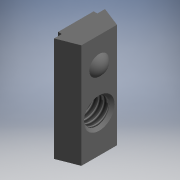
# Autodesk Inventor part: HNTP5-5_app
Saved by Autodesk Inventor 2017.3 (Build 213256000, 256)
## iProperties
Part Number: HNTP5-5_app
Material: Generic
Catalog Web Link: www.cadenas.de
Description: HNTP, HNTPV, HNTPZ, SHNTP_app-Post-Assembly Fitting Spring Nuts For Aluminum Frames
Vendor: MISUMI
Document SubType Name: Modeling
Designer: partserver
Manufacturer: MISUMI
Mass: 0.392555 g
Surface Area: 4.47403 cm^2
Volume: 0.392555 cm^3
Density: 1 g/cm^3
Appearance: PSOLRGB-128-128-128
Category: PARTsolutions
Company: MISUMI
Title: HNTP5-5
Author: Cadenas PARTsolutions
Comments: Post-Assembly Fitting Spring Nuts For Aluminum Frames
PSOL_IDENT_0: {$CADENAS_DATA\23d-libs\misumi\metric\38_al_extrusions_blackets\nuts\shntp.prj},188 {VTYP=3D},{NB=HN
PSOL_IDENT_1: TP5-5_app},{LINA=HNTP5-5},{NN=HNTP, HNTPV, HNTPZ, SHNTP_app},{DATE=28.07.2021 09:30:14},{GEOMDATE=07
PSOL_IDENT_2: .03.2017 06:48:08},{VERSION=},{LINEID=10},{WBVAR=MATB,M},{WBNUMERIC=M}  {NB=HNTP5-5_app},{LINA=HNTP5
PSOL_IDENT_3: -5},{KT=DUMMY},{PN=HNTP5-5},{MATB=HNTP},{MATBALL=304 Stainless Steel},{MATS=SWP-A},{ST=Trivalent Chr
PSOL_IDENT_4: omate},{NO=5},{M=5},{MALG=3,4,5},{AFS=HFS5},{A=5.8},{B=8.3},{E=3.2},{T=3.8},{L=17},{L1=6.0},{TT=6.8}
PSOL_IDENT_5: ,{L11=4}
NB: HNTP5-5_app
NN: HNTP, HNTPV, HNTPZ, SHNTP_app
NT: Post-Assembly Fitting Spring Nuts For Aluminum Frames
NBSYN: $PN._app
LINA: HNTP5-5
CATALOG: Misumi
PN: HNTP5-5
MATB: 1010 Carbon Steel Equivalent
MATBALL: 304 Stainless Steel
MATS: SWP-A
ST: Trivalent Chromate Plating
NO: 5
M: 5
A: 5.8
B: 8.3
E: 3.2
T: 3.8
L: 17
L1: 6
TT: 6.8
SUPPLIER: MISUMI
ARTICLENO: HNTP5-5_app
BOMINFO: HNTP5-5
CREATOR: CADENAS GmbH
Autodesk Inventor part; units mm, degrees
sketch "Sketch_1" plane through (0, 0, 0) normal (0, 0, 1) x (1, 0, 0)
  line L0 (0, -2.9) -> (3.2, -4.15)
  line L1 (3.2, -4.15) -> (3.2, -2.9)
  line L2 (3.2, -2.9) -> (3.8, -2.9)
  line L3 (3.8, -2.9) -> (3.8, 2.9)
  line L4 (3.8, 2.9) -> (3.2, 2.9)
  line L5 (3.2, 2.9) -> (3.2, 4.15)
  line L6 (3.2, 4.15) -> (0, 2.9)
  line L7 (0, 2.9) -> (0, -2.9)
  constraints: 16 end point
extrude "Extrusion1" add sketch "Sketch_1" along normal mid plane 17
sketch "Sketch_2" plane through (0, 0, 2.5) normal (0, 0, 1) x (1, 0, 0)
  line L0 (3.8, 0) -> (0, 0)
  line L1 (0, 0) -> (0, 2.5)
  line L2 (0, 2.5) -> (0.433, 2.067)
  line L3 (0.433, 2.067) -> (3.367, 2.067)
  line L4 (3.367, 2.067) -> (3.8, 2.5)
  line L5 (3.8, 2.5) -> (3.8, 0)
  line L6 (3.8, 0) -> (0, 0)
  constraints: 14 end point
revolve "Revolution1" cut sketch "Sketch_2" angle 360 about axis through (3.8, 0, 2.5) along (1, 0, 0)
thread "Thread1" size "M5x0.8" class "6H" standard "ISO Metric profile" full length
sketch "Sketch_3" plane through (0, 0, -4.25) normal (0, 0, 1) x (1, 0, 0)
  line L0 (1.2, 3.2) -> (1.2, -3.2)
  arc A0 (1.2, 2) -> (1.2, -2) centre (1.2, 0) ccw
  line L1 (1.2, 2) -> (1.2, -2)
  constraints: 4 end point, 2 point on circle, 1 centre point
revolve "Revolution2" add sketch "Sketch_3" angle 360 about axis through (1.2, 3.2, -4.25) along (0, 1, 0)
ref_plane "nut1_to_bolt1_XY" through (3.8, 0, 2.5) normal (1, 0, 0) x (0, 0, -1)
ref_plane "nut1_to_bolt1_YZ" through (3.8, 0, 2.5) normal (0, 0, -1) x (0, 1, 0)
ref_plane "nut1_to_bolt1_ZX" through (3.8, 0, 2.5) normal (0, 1, 0) x (1, 0, 0)
ref_plane "nut_to_bolt_XY" through (0, 0, 2.5) normal (1, 0, 0) x (0, 0, -1)
ref_plane "nut_to_bolt_YZ" through (0, 0, 2.5) normal (0, 0, -1) x (0, 1, 0)
ref_plane "nut_to_bolt_ZX" through (0, 0, 2.5) normal (0, 1, 0) x (1, 0, 0)
ref_plane "to_frames_XY" through (3.2, 0, 2.5) normal (1, 0, 0) x (0, 0, -1)
ref_plane "to_frames_YZ" through (3.2, 0, 2.5) normal (0, 0, -1) x (0, 1, 0)
ref_plane "to_frames_ZX" through (3.2, 0, 2.5) normal (0, 1, 0) x (1, 0, 0)
body "Solid1"
